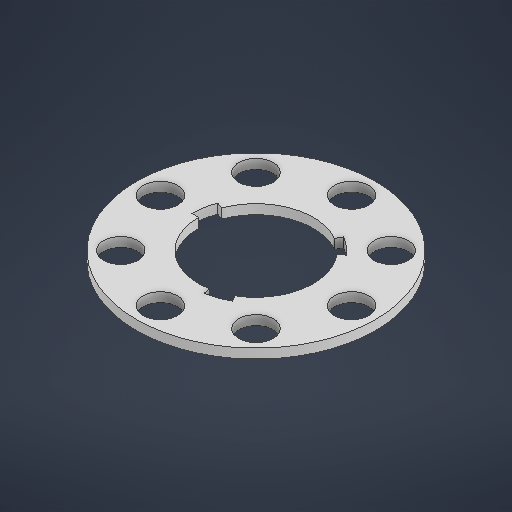
# Autodesk Inventor part: Part1
Saved by Autodesk Inventor 2026.2 (Build 302298000, 298)
## iProperties
Created: 2026-01-26
Part Number: Part1
Material: Generic
Document SubType Name: Modeling
Designer: Cobble
Density: 1 g/cm^3
Appearance: Default
Author: Cobble
Autodesk Inventor part; units mm, degrees
ref_plane "YZ Plane" through (0, 0, 0) normal (1, 0, 0) x (0, 1, 0)
ref_plane "XZ Plane" through (0, 0, 0) normal (0, 1, 0) x (-1, 0, 0)
ref_plane "XY Plane" through (0, 0, 0) normal (0, 0, 1) x (1, 0, 0)
sketch "Sketch1" plane through (0, 0, 0) normal (0, 0, 1) x (1, 0, 0)
  circle A0 centre (0, 0) radius 100 construction
  circle A1 centre (-100, 0) radius 18
  circle A2 centre (-70.7107, -70.7107) radius 18
  circle A3 centre (0, -100) radius 18
  circle A4 centre (70.7107, -70.7107) radius 18
  circle A5 centre (100, 0) radius 18
  circle A6 centre (70.7107, 70.7107) radius 18
  circle A7 centre (0, 100) radius 18
  circle A8 centre (-70.7107, 70.7107) radius 18
  circle A9 centre (0, 0) radius 125
  circle A10 centre (0, 0) radius 75
  circle A11 centre (0, 0) radius 67.5 construction
  circle A12 centre (0, 0) radius 67
  circle A13 centre (0, 0) radius 60
  line L0 (0, 0) -> (-67, 0)
  line L1 (0, 0) -> (-2.0269, 0)
  line L2 (0, 0) -> (-62.9594, 22.9153)
  line L3 (0, 0) -> (67, 0) construction
  line L4 (0, 0) -> (33.5, -58.0237)
  line L5 (0, 0) -> (11.6344, -65.9821)
  line L6 (0, 0) -> (33.5, 58.0237)
  line L7 (0, 0) -> (51.325, 43.0668)
  point P0 (1.0135, -1.7554)
  point P1 (1.0135, 1.7554)
  point P2 (10.4189, -59.0885)
  point P3 (-60, 0)
  point P4 (-56.3816, 20.5212)
  point P5 (30, 51.9615)
  point P6 (45.9627, 38.5673)
  point P7 (30, -51.9615)
  dimension "d0" = 200
  dimension "d1" = 36
  dimension "d4" = 360
  dimension "d6" = 250
  dimension "d7" = 150
  dimension "d10" = 135
  dimension "d11" = 134
  dimension "d12" = 120
  dimension "d13" = 160
  dimension "d16" = 360
  constraints: 16 end point, 13 centre point, 6 coincident, 3 point on line, 2 horizontal, 2 point on circle, 1 equal length, 1 horizontal alignment, 38 other
  measures "d1" diameter of A1
  measures "d6" diameter of A9
  measures "d7" diameter of A10
  measures "d10" diameter of A11
  measures "d11" diameter of A12
  measures "d12" diameter of A13
  measures "d13" angle of L3 L2
extrude "Extrusion1" add sketch "Sketch1" along normal blind 10 contours A9 | A10 | A12 L4 A13 L7 | L6 A13 L2 A12 | A12 L0 A13 L5
equation "\"d0\" = OuterRadius"
equation "\"OuterRadius\" = 200"
body "Solid1"
